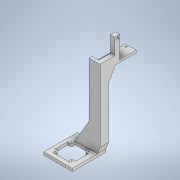
# Autodesk Inventor part: camera_mount_v2
Saved by Autodesk Inventor 2022 (Build 260153000, 153)
## iProperties
Created: 2022-06-05
Part Number: camera_mount_v2
Material: Generic
Document SubType Name: Modeling
Designer: kylem
Density: 1 g/cm^3
Appearance: Default
Author: kylem
Autodesk Inventor part; units mm, degrees
ref_plane "YZ Plane" through (0, 0, 0) normal (1, 0, 0) x (0, 1, 0)
ref_plane "XZ Plane" through (0, 0, 0) normal (0, 1, 0) x (-1, 0, 0)
ref_plane "XY Plane" through (0, 0, 0) normal (0, 0, 1) x (1, 0, 0)
sketch "Sketch1" plane through (0, 0, 0) normal (0, 1, 0) x (-1, 0, 0)
  line L0 (0, 0) -> (13, 0)
  line L1 (13, 0) -> (13, -44)
  line L2 (13, -44) -> (0, -44)
  line L3 (0, -44) -> (0, 0)
  line L4 (13, 0) -> (13, -6)
  line L5 (13, -6) -> (7.5, -6)
  line L6 (7.5, -6) -> (7.5, -40)
  circle A0 centre (7.5, -6) radius 1.65
  circle A1 centre (7.5, -40) radius 1.65
  dimension "d0" = 13
  dimension "d1" = 44
  dimension "d2" = 6
  dimension "d3" = 5.5
  dimension "d4" = 34
  dimension "d5" = 3.3
  dimension "d6" = 3.3
  constraints: 14 end point, 3 parallel, 2 centre point, 2 coincident, 2 perpendicular, 1 horizontal, 1 point on line
  measures "d0" distance of L1.end L2.end
  measures "d1" distance of L0.end L1.end
  measures "d2" distance of L0.end L4.end
  measures "d3" distance of L4.end L5.end
  measures "d4" distance of L5.end L6.end
  measures "d5" diameter of A0
  measures "d6" diameter of A1
extrude "Extrusion1" add sketch "Sketch1" along normal blind 5
sketch "Sketch2" plane through (0, 0, 0) normal (1, 0, 0) x (0, 0, -1)
  line L0 (0, 5) -> (44, 5) projected
  line L1 (0, 5) -> (44, 5)
  line L2 (44, 5) -> (44, 50)
  line L3 (44, 50) -> (0, 50)
  line L4 (0, 50) -> (0, 5)
  line L5 (0, 0) -> (44, 0)
  line L6 (44, 0) -> (44, 5)
  line L7 (44, 5) -> (0, 5)
  line L8 (0, 5) -> (0, 0)
  line L9 (0, 50) -> (10, 50)
  line L10 (10, 50) -> (10, 5)
  line L11 (10, 5) -> (0, 5)
  line L12 (0, 5) -> (0, 50)
  dimension "d9" = 44
  dimension "d10" = 45
  dimension "d11" = 10
  constraints: 24 end point, 6 parallel, 3 horizontal, 3 perpendicular, 1 point on line
  measures "d9" distance of L3.end L2.end
  measures "d10" distance of L2.end L1.end
  measures "d11" distance of L10.end L11.end
extrude "Extrusion2" add sketch "Sketch2" along normal blind 4 contours L4 L3 L10 L0 | L0 L6 L5 L8
sketch "Sketch3" plane through (4, 0, 0) normal (1, 0, 0) x (0, 0, -1)
  line L0 (44, 5) -> (10, 5) projected
  line L1 (10, 5) -> (10, 45)
  line L2 (10, 5) -> (10, 50) projected
  line L3 (0, 50) -> (0, 5) projected
  line L4 (0, 45) -> (4.4, 45)
  line L5 (6, 45) -> (6, 46.5)
  line L6 (6, 45) -> (6, 43.5)
  line L7 (4.4, 46.5) -> (4.4, 43.5)
  line L8 (7.6, 46.5) -> (7.6, 43.5)
  arc A0 (5.4432, 45) -> (6, 44.9) centre (6, 46.5) ccw
  arc A1 (6.5568, 45) -> (4.4, 46.5) centre (6, 46.5) ccw
  line L9 (10, 45) -> (6.5568, 45)
  line L10 (5.4432, 45) -> (0, 45)
  arc A2 (6, 45.1) -> (5.4432, 45) centre (6, 43.5) ccw
  arc A3 (4.4, 43.5) -> (7.6, 43.5) centre (6, 43.5) ccw
  point P0 (0, 0)
  dimension "d14" = 40
  dimension "d15" = 6
  dimension "d16" = 1.5
  dimension "d17" = 1.5
  constraints: 16 end point, 9 point on circle, 4 centre point, 4 tangent, 3 point on line, 2 coincident, 2 perpendicular, 2 vertical, 1 midpoint
  measures "d14" distance of L0.end L1.end
  measures "d15" distance of L4.start L5.start
  measures "d16" distance of L5.start L5.end
  measures "d17" distance of L5.start L6.end
extrude "Extrusion3" cut sketch "Sketch3" against normal blind 4 contours L6 A0 A2 L5 | A1 L9 L8 A3 L7 | L8 L9 A1
sketch "Sketch4" plane through (-13, 0, 0) normal (0, 0, 1) x (1, 0, 0)
  line L0 (0, 0) -> (17, 0) projected
  line L1 (17, 0) -> (17, 5) projected
  line L2 (0, 0) -> (17, 0)
  line L3 (17, 0) -> (17, 5)
  line L4 (17, 5) -> (0, 5)
  line L5 (0, 5) -> (0, 0)
  line L6 (13, 50) -> (13, 5) projected
  line L7 (17, 0) -> (13, 0)
  line L8 (13, 0) -> (13, 17)
  line L9 (13, 17) -> (17, 17)
  line L10 (17, 17) -> (17, 0)
  dimension "d22" = 17
  constraints: 16 end point, 4 parallel, 2 horizontal, 2 perpendicular, 1 point on line
  measures "d22" distance of L7.end L8.end
extrude "Extrusion4" add sketch "Sketch4" along normal blind 30
sketch "Sketch5" plane through (0, 0, 0) normal (0, -1, 0) x (1, 0, 0)
  line L0 (-13, -44) -> (-13, 30) projected
  line L1 (-13, 30) -> (4, 30)
  line L2 (4, 30) -> (4, 13)
  line L3 (4, 13) -> (-13, 13)
  line L4 (-13, 13) -> (-13, 30)
  point P0 (0, 0)
  dimension "d25" = 17
  dimension "d26" = 17
  constraints: 8 end point, 2 parallel, 1 horizontal, 1 perpendicular
  measures "d25" distance of L2.end L3.end
  measures "d26" distance of L1.end L2.end
extrude "Extrusion5" add sketch "Sketch5" along normal blind 150
sketch "Sketch7" plane through (0, -150, 0) normal (0, -1, 0) x (1, 0, 0)
  line L0 (4, 13) -> (-13, 13) projected
  line L1 (0, 30) -> (0, -10) projected
  line L2 (0, 13) -> (0, 30)
  line L3 (0, 30) -> (0, 52.6)
  circle A0 centre (-36, 52.6) radius 9
  line L4 (-36, 52.6) -> (-36, 36.6)
  line L5 (-36, 36.6) -> (-20, 36.6)
  line L6 (-36, 52.6) -> (-36, 68.6)
  line L7 (-36, 68.6) -> (-52, 68.6)
  line L8 (-52, 68.6) -> (-20, 68.6)
  line L9 (-20, 68.6) -> (-20, 36.6)
  line L10 (-20, 36.6) -> (-52, 36.6)
  line L11 (-52, 36.6) -> (-52, 68.6)
  circle A1 centre (-20, 68.6) radius 1.1
  circle A2 centre (-20, 36.6) radius 1.1
  circle A3 centre (-52, 36.6) radius 1.1
  circle A4 centre (-52, 68.6) radius 1.1
  circle A5 centre (-20, 68.6) radius 4
  circle A6 centre (-20, 36.6) radius 4
  line L12 (-52, 65.6) -> (-52, 70.6)
  line L13 (-52, 36.6) -> (-52, 42.6)
  circle A7 centre (-52, 68.6) radius 4
  circle A8 centre (-52, 36.6) radius 4
  point P0 (0, 0)
  point P1 (-20, 64.6)
  point P2 (-20, 40.6)
  dimension "d29" = 22.6
  dimension "d31" = 18
  dimension "d32" = 16
  dimension "d33" = 16
  dimension "d34" = 16
  dimension "d35" = 16
  dimension "d36" = 2.2
  dimension "d37" = 2.2
  dimension "d39" = 2.2
  dimension "d40" = 8
  dimension "d43" = 8
  dimension "d49" = 8
  dimension "d50" = 8
  constraints: 24 end point, 9 centre point, 8 coincident, 3 perpendicular, 3 point on line, 2 parallel, 2 vertical, 1 collinear, 1 horizontal
  measures "d29" distance of L1.start L3.end
  measures "d31" diameter of A0
  measures "d32" distance of L4.start L4.end
  measures "d33" distance of L4.end L5.end
  measures "d34" distance of L4.start L6.end
  measures "d35" distance of L6.end L7.end
  measures "d36" diameter of A1
  measures "d37" diameter of A2
  measures "d39" diameter of A4
  measures "d40" diameter of A5
  measures "d43" diameter of A6
  measures "d49" diameter of A7
  measures "d50" diameter of A8
sketch "Sketch14" plane through (0, -150, 0) normal (0, -1, 0) x (1, 0, 0)
  line L0 (4, 13) -> (4, 30) projected
  line L1 (4, 13) -> (4, 52.6)
  line L2 (4, 52.6) -> (-26.5, 52.6)
  line L3 (-26.5, 52.6) -> (-26.5, 35.35)
  line L4 (-26.5, 35.35) -> (-9.25, 35.35)
  line L5 (-26.5, 52.6) -> (-43.75, 52.6)
  line L6 (-43.75, 52.6) -> (-43.75, 69.85)
  line L7 (-43.75, 69.85) -> (-9.25, 69.85)
  line L8 (-9.25, 69.85) -> (-9.25, 35.35)
  line L9 (-9.25, 35.35) -> (-43.75, 35.35)
  line L10 (-43.75, 35.35) -> (-43.75, 69.85)
  circle A0 centre (-43.75, 69.85) radius 0.95
  circle A1 centre (-9.25, 69.85) radius 0.95
  circle A2 centre (-9.25, 35.35) radius 0.95
  circle A3 centre (-43.75, 35.35) radius 0.95
  circle A4 centre (-43.75, 69.85) radius 4
  circle A5 centre (-9.25, 69.85) radius 4
  circle A6 centre (-9.25, 35.35) radius 4
  circle A7 centre (-43.75, 35.35) radius 4
  point P0 (0, 0)
  dimension "d91" = 39.6
  dimension "d92" = 30.5
  dimension "d93" = 17.25
  dimension "d94" = 17.25
  dimension "d95" = 17.25
  dimension "d96" = 17.25
  dimension "d97" = 1.9
  dimension "d98" = 1.9
  dimension "d99" = 1.9
  dimension "d100" = 1.9
  dimension "d101" = 8
  dimension "d102" = 8
  dimension "d103" = 8
  dimension "d104" = 8
  constraints: 20 end point, 8 centre point, 8 coincident, 4 perpendicular, 2 horizontal, 2 parallel, 1 collinear, 1 vertical
  measures "d91" distance of L0.start L1.end
  measures "d92" distance of L1.end L2.end
  measures "d93" distance of L2.end L3.end
  measures "d94" distance of L3.end L4.end
  measures "d95" distance of L2.end L5.end
  measures "d96" distance of L5.end L6.end
  measures "d97" diameter of A0
  measures "d98" diameter of A1
  measures "d99" diameter of A2
  measures "d100" diameter of A3
  measures "d101" diameter of A4
  measures "d102" diameter of A5
  measures "d103" diameter of A6
  measures "d104" diameter of A7
extrude "Extrusion14" add sketch "Sketch14" against normal blind 6 contours A5 L7 A1 L8 | L8 A1 L7 A5 | A6 L4 A2 L8 | L8 A2 L4 A6 | A7 L10 A3 L9 | L9 A3 L10 A7 | A4 L7 A0 L6 | L6 A0 L7 A4
sketch "Sketch15" plane through (-9.25, -150, 69.85) normal (0, -1, 0) x (1, 0, 0)
  circle A0 centre (0, 0) radius 4 projected
  line L0 (0, 4) -> (10, 4)
  line L1 (10, 4) -> (10, -4)
  line L2 (10, -4) -> (0, -4)
  line L3 (0, -4) -> (0, 4)
  circle A1 centre (0, -34.5) radius 4 projected
  line L4 (0, -30.5) -> (10, -30.5)
  line L5 (10, -30.5) -> (10, -38.5)
  line L6 (10, -38.5) -> (0, -38.5)
  line L7 (0, -38.5) -> (0, -30.5)
  circle A2 centre (-34.5, -34.5) radius 4 projected
  line L8 (-34.5, -38.5) -> (-44.5, -38.5)
  line L9 (-44.5, -38.5) -> (-44.5, -30.5)
  line L10 (-44.5, -30.5) -> (-34.5, -30.5)
  line L11 (-34.5, -30.5) -> (-34.5, -38.5)
  circle A3 centre (-34.5, 0) radius 4 projected
  line L12 (-34.5, -4) -> (-44.5, -4)
  line L13 (-44.5, -4) -> (-44.5, 4)
  line L14 (-44.5, 4) -> (-34.5, 4)
  line L15 (-34.5, 4) -> (-34.5, -4)
  line L16 (-44.5, 4) -> (-38.5, 4)
  line L17 (-38.5, 4) -> (-38.5, -38.5)
  line L18 (-38.5, -38.5) -> (-44.5, -38.5)
  line L19 (-44.5, -38.5) -> (-44.5, 4)
  line L20 (10, 4) -> (4, 4)
  line L21 (4, 4) -> (4, -38.5)
  line L22 (4, -38.5) -> (10, -38.5)
  line L23 (10, -38.5) -> (10, 4)
  point P0 (9.25, -69.85)
  point P1 (-38.5, -4)
  point P2 (-34.5, 4)
  point P3 (-34.5, -30.5)
  point P4 (-38.5, -30.5)
  point P5 (0, -4)
  point P6 (4, -4)
  point P7 (4, -30.5)
  point P8 (0, -38.5)
  point P9 (10, -4)
  dimension "d107" = 10
  dimension "d108" = 8
  dimension "d109" = 10
  dimension "d110" = 8
  dimension "d111" = 10
  dimension "d112" = 8
  dimension "d113" = 10
  dimension "d114" = 8
  dimension "d115" = 6
  dimension "d116" = 6
  constraints: 48 end point, 12 parallel, 6 horizontal, 6 perpendicular, 5 point on line, 8 other
  measures "d107" distance of L1.end L2.end
  measures "d108" distance of L0.end L1.end
  measures "d109" distance of L5.end L6.end
  measures "d110" distance of L4.end L5.end
  measures "d111" distance of L9.end L10.end
  measures "d112" distance of L8.end L9.end
  measures "d113" distance of L13.end L14.end
  measures "d114" distance of L12.end L13.end
  measures "d115" distance of L17.end L18.end
  measures "d116" distance of L22.end L21.end
extrude "Extrusion15" add sketch "Sketch15" against normal blind 6 contours L21 L2 A0 | A0 L0 L21 | L21 L0 L1 L2 | L2 L23 L4 L21 | L21 A1 L4 | L4 L5 L6 L21 | L21 L6 A1 | A2 L17 L10 | L8 L17 A2 | L17 L8 L9 L10 | L10 L19 L12 L17 | L17 A3 L12 | L12 L13 L14 L17 | L17 L14 A3
sketch "Sketch16" plane through (0, -150, 0) normal (0, -1, 0) x (1, 0, 0)
  line L0 (0.75, 73.85) -> (0.75, 31.35) projected
  line L1 (0.75, 73.85) -> (-51.25, 73.85)
  line L2 (-51.25, 73.85) -> (-51.25, 81.85)
  line L3 (-51.25, 81.85) -> (0.75, 81.85)
  line L4 (0.75, 81.85) -> (0.75, 73.85)
  line L5 (0.75, 31.35) -> (-9.25, 31.35) projected
  line L6 (0.75, 31.35) -> (-51.25, 31.35)
  line L7 (-51.25, 31.35) -> (-51.25, 23.35)
  line L8 (-51.25, 23.35) -> (0.75, 23.35)
  line L9 (0.75, 23.35) -> (0.75, 31.35)
  point P0 (0, 0)
  dimension "d119" = 8
  dimension "d120" = 8
  constraints: 16 end point, 4 parallel, 2 horizontal, 2 perpendicular
  measures "d119" distance of L1.end L2.end
  measures "d120" distance of L7.end L6.end
extrude "Extrusion16" add sketch "Sketch16" against normal blind 6
sketch "Sketch17" plane through (0, -144, 0) normal (0, 1, 0) x (1, 0, 0)
  line L0 (0.75, -81.85) -> (0.75, -30) projected
  line L1 (4, -30) -> (0, -30) projected
  line L2 (0.75, -81.85) -> (4, -81.85)
  line L3 (4, -81.85) -> (4, -30)
  line L4 (4, -30) -> (0.75, -30)
  line L5 (0.75, -30) -> (0.75, -81.85)
  line L6 (-51.25, -23.35) -> (-51.25, -81.85) projected
  line L7 (-51.25, -23.35) -> (-13, -23.35)
  line L8 (-13, -23.35) -> (-13, -13)
  line L9 (-13, -13) -> (-51.25, -13)
  line L10 (-51.25, -13) -> (-51.25, -23.35)
  point P0 (0, 0)
  point P1 (0.75, -30)
  point P2 (0.75, -30)
  constraints: 16 end point, 4 parallel, 2 horizontal, 2 perpendicular
extrude "Extrusion17" add sketch "Sketch17" against normal blind 6
chamfer "Chamfer4" distance 50 angle 30 1 edges at (-13, -144, 21.5) measured on face at (-13, -143.5, 21.5)
chamfer "Chamfer5" distance 25 angle 30 1 edges at (-4.5, 0, 13) measured on face at (-4.5, -0.5, 13)
sketch "Sketch19" plane through (-13, 0, 30) normal (0, 0, 1) x (1, 0, 0)
  line L0 (13, 17) -> (13, 5) projected
  line L1 (0, 0) -> (0, 5) projected
  line L2 (13, 17) -> (0, 17)
  line L3 (0, 17) -> (0, 5)
  line L4 (0, 5) -> (13, 5)
  line L5 (13, 5) -> (13, 17)
  point P0 (13, 0)
  constraints: 8 end point, 2 parallel, 1 horizontal, 1 perpendicular
extrude "Extrusion18" add sketch "Sketch19" against normal blind 6
sketch "Sketch20" plane through (-51.25, -150, 13) normal (-1, 0, 0) x (0, 0, 1)
  line L0 (0, 125) -> (0, 0) projected
  line L1 (60.85, 6) -> (68.85, 6) projected
  line L2 (0, 0) -> (68.85, 0)
  line L3 (68.85, 0) -> (68.85, 6)
  line L4 (68.85, 6) -> (0, 6)
  line L5 (0, 6) -> (0, 0)
  point P0 (-13, 150)
  constraints: 8 end point, 2 parallel, 1 horizontal, 1 perpendicular
extrude "Extrusion19" add sketch "Sketch20" along normal blind 3
sketch "Sketch21" plane through (0, 0, 0) normal (-1, 0, 0) x (0, 0, 1)
  line L0 (-10, 5) -> (-10, 50) projected
  line L1 (24, 5) -> (-10, 5) projected
  line L2 (-10, 50) -> (24, 50)
  line L3 (24, 50) -> (24, 5)
  line L4 (24, 5) -> (-10, 5)
  line L5 (-10, 5) -> (-10, 50)
  point P0 (0, 0)
  constraints: 8 end point, 2 parallel, 1 horizontal, 1 perpendicular
extrude "Extrusion20" cut sketch "Sketch21" against normal blind 0.2
chamfer "Chamfer6" distance 2 angle 15 1 edges at (-10.2, -150, 69.85) measured on face at (-10.2, -149.5, 69.85)
chamfer "Chamfer7" distance 2 angle 15 1 edges at (-10.2, -150, 35.35) measured on face at (-10.2, -149.5, 35.35)
chamfer "Chamfer8" distance 2 angle 15 1 edges at (-44.7, -150, 35.35) measured on face at (-44.7, -149.5, 35.35)
chamfer "Chamfer9" distance 2 angle 15 1 edges at (-44.7, -150, 69.85) measured on face at (-44.7, -149.5, 69.85)
sketch "Sketch22" plane through (4, 0, 0) normal (1, 0, 0) x (0, 0, -1)
  line L0 (44, 0) -> (1.4338, 0) projected
  line L1 (-30, 17) -> (-30, -144) projected
  line L2 (44, 0) -> (-30, 0)
  line L3 (-30, 0) -> (-30, 17)
  line L4 (-30, 17) -> (44, 17)
  line L5 (44, 17) -> (44, 0)
  line L6 (10, 50) -> (0, 50) projected
  line L7 (10, 50) -> (0, 50)
  line L8 (0, 50) -> (0, 0)
  line L9 (0, 0) -> (10, 0)
  line L10 (10, 0) -> (10, 50)
  line L11 (10, 5) -> (10, 50) projected
  line L12 (44, 17) -> (10, 17)
  line L13 (10, 17) -> (10, 5)
  line L14 (10, 5) -> (44, 5)
  line L15 (44, 5) -> (44, 17)
  arc A0 (4.4, 43.5) -> (7.6, 43.5) centre (6, 43.5) ccw projected
  circle A1 centre (6, 43.5) radius 1.6
  arc A2 (7.6, 46.5) -> (4.4, 46.5) centre (6, 46.5) ccw projected
  circle A3 centre (6, 46.5) radius 1.6
  line L16 (7.6, 46.5) -> (7.6, 43.5) projected
  line L17 (7.6, 46.5) -> (7.6, 43.5)
  line L18 (7.6, 43.5) -> (4.4, 43.5)
  line L19 (4.4, 43.5) -> (4.4, 46.5) projected
  line L20 (4.4, 46.5) -> (4.4, 43.5)
  point P0 (0, 17)
  point P1 (1.4338, 0)
  constraints: 30 end point, 8 equal length, 4 perpendicular, 3 horizontal, 3 vertical, 2 coincident, 2 horizontal alignment, 1 tangent, 4 other
extrude "Extrusion21" add sketch "Sketch22" along normal blind 5 contours L0 L10 L14 L5 | L0 L2 L8 L4 L10 | L2 L1 L4 L8 | L4 L8 L6 L10
sketch "Sketch23" plane through (4, 0, 0) normal (1, 0, 0) x (0, 0, -1)
  line L0 (-13, -25) -> (-13, -94) projected
  line L1 (-13, -25) -> (1.4338, 0) projected
  line L2 (-13, -25) -> (1.4338, 0)
  line L3 (-30, 0) -> (44, 0) projected
  line L4 (1.4338, 0) -> (-30, 0)
  line L5 (-30, 0) -> (-30, -144) projected
  line L6 (-30, 0) -> (-30, -144)
  line L7 (-81.85, -144) -> (-13, -144) projected
  line L8 (-30, -144) -> (-13, -144)
  line L9 (-13, -144) -> (-13, -25)
  point P0 (0, 0)
  constraints: 10 end point, 3 collinear, 2 perpendicular
extrude "Extrusion22" add sketch "Sketch23" along normal blind 5
chamfer "Chamfer10" distance 13.737 angle 20 1 edges at (9, -144, 21.5) measured on face at (9, -143.5, 21.5)
body "Solid1"
